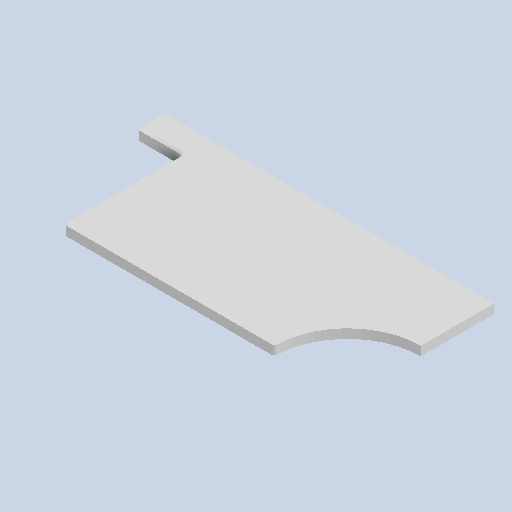
# Autodesk Inventor part: Lado Esquerdo Mesa
Saved by Autodesk Inventor 2025.2 (Build 292293000, 293)
## iProperties
Created: 2025-04-07
Part Number: Lado Esquerdo Mesa
Material: Genérico
Document SubType Name: Modeling
Designer: kenay
Density: 1 g/cm^3
Appearance: Padrão
Author: kenay
Autodesk Inventor part; units mm, degrees
ref_plane "YZ Plane" through (0, 0, 0) normal (1, 0, 0) x (0, 1, 0)
ref_plane "XZ Plane" through (0, 0, 0) normal (0, 1, 0) x (-1, 0, 0)
ref_plane "XY Plane" through (0, 0, 0) normal (0, 0, 1) x (1, 0, 0)
sketch "Esboço1" plane through (0, 0, 0) normal (0, 1, 0) x (-1, 0, 0)
  line L0 (-900, 400) -> (900, 400) construction
  line L1 (900, 400) -> (900, -400) construction
  line L2 (900, -400) -> (-900, -400) construction
  line L3 (-900, -400) -> (-900, 400) construction
  line L4 (-900, 400) -> (900, -400) construction
  line L5 (900, 400) -> (-900, -400) construction
  line L6 (900, -250) -> (650, -250) construction
  line L7 (650, -250) -> (650, 400) construction
  arc A0 (885, -400) -> (900, -385) centre (885, -385) ccw
  arc A1 (650, -235) -> (665, -250) centre (665, -235) ccw
  line L8 (885, -400) -> (-900, -400)
  line L9 (900, -385) -> (900, -250) construction
  line L10 (900, -250) -> (665, -250) construction
  line L11 (-900, -400) -> (-1700, -400) construction
  line L12 (-1700, -400) -> (-1700, 1400) construction
  line L13 (-1700, 1400) -> (-900, 1400) construction
  line L14 (-900, 1400) -> (-900, -400) construction
  circle A2 centre (-900, 400) radius 400 construction
  line L15 (900, 0) -> (-900, 0) construction
  line L16 (-1300, 1400) -> (-1300, -404.7673) construction
  arc A3 (-485.2712, 400) -> (-500.2614, 385.5422) centre (-485.2712, 385) ccw
  line L17 (650, -235) -> (650, 385)
  arc A4 (650, 385) -> (635, 400) centre (635, 385) ccw
  line L18 (635, 400) -> (-485.2712, 400)
  arc A5 (-900, 0) -> (-500.2614, 385.5422) centre (-900, 400) ccw
  line L19 (-900, -400) -> (-900, 0)
  arc A6 (900, -265) -> (885, -250) centre (885, -265) ccw
  line L20 (900, -265) -> (900, -385)
  line L21 (885, -250) -> (665, -250)
  point P0 (0, 0)
  dimension "d11" = 800
  dimension "d0" = 800
  dimension "d1" = 1800
  dimension "d3" = 650
  dimension "d5" = 15
  dimension "d6" = 800
  dimension "d7" = 1800
  dimension "d9" = 250
  dimension "d13" = 400
  dimension "d14" = 400
  dimension "d15" = 400
  constraints: 44 end point, 12 point on circle, 10 point on line, 9 tangent, 6 centre point, 5 horizontal, 4 equal radius, 4 midpoint, 4 parallel, 4 perpendicular, 2 vertical, 5 other
  measures "d0" distance between parallel lines of L0 L2
  measures "d1" distance between parallel lines of L3 L1
  measures "d3" distance of L6.end L7.end
  measures "d5" radius of A0
  measures "d6" distance of L12.end L13.end
  measures "d7" distance of L11.end L12.end
  measures "d9" distance between parallel lines of L1 L7
  measures "d13" radius of A5
  measures "d14" distance between parallel lines of L12 L16
  measures "d15" distance from line of L19.end L11
sketch "Esboço3" plane through (0, 0, 0) normal (0, 1, 0) x (-1, 0, 0)
  line L0 (-900, 400) -> (900, 400) construction
  line L1 (900, 400) -> (900, -400) construction
  line L2 (900, -400) -> (-900, -400) construction
  line L3 (-900, -400) -> (-900, 400) construction
  line L4 (-900, 400) -> (900, -400) construction
  line L5 (900, 400) -> (-900, -400) construction
  arc A0 (-900, -350) -> (-850, -400) centre (-850, -350) ccw
  arc A1 (850, -400) -> (900, -350) centre (850, -350) ccw
  line L6 (900, 0) -> (-900, 0) construction
  line L7 (700, 400) -> (700, 0) construction
  line L8 (850, -400) -> (-850, -400)
  line L9 (900, -350) -> (900, 400)
  line L10 (-900, -350) -> (-900, -350)
  line L11 (-900, -309.491) -> (-900, -350)
  arc A2 (-850, 400) -> (-900, 350) centre (-850, 350) ccw
  line L12 (-900, -309.491) -> (-900, 350)
  circle A3 centre (300, 400) radius 400 construction
  arc A4 (-97.5232, 355.5556) -> (-147.2136, 400) centre (-147.2136, 350) ccw
  line L13 (900, 400) -> (700, 400)
  line L14 (-147.2136, 400) -> (-850, 400)
  arc A5 (-97.5232, 355.5556) -> (700, 400) centre (300, 400) ccw
  point P0 (0, 0)
  point P1 (-498.6068, 400)
  dimension "d16" = 1800
  dimension "d17" = 800
  dimension "d19" = 200
  dimension "d20" = 50
  dimension "d21" = 800
  constraints: 30 end point, 12 point on circle, 12 point on line, 10 tangent, 6 centre point, 5 midpoint, 3 equal radius, 2 horizontal, 2 parallel, 2 perpendicular
  measures "d16" distance of L1.end L2.end
  measures "d17" distance of L0.end L1.end
  measures "d19" distance between parallel lines of L1 L7
  measures "d20" radius of A1
  measures "d21" diameter of A3
extrude "Extrusão1" add sketch "Esboço1" along normal mid plane 50
equation "\"d6\" = d0"
equation "\"d7\" = d1"
